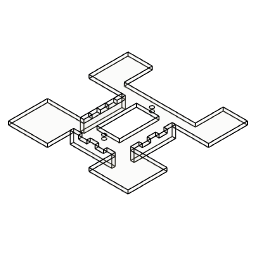
servo support (Autodesk Fusion 360 design; units mm, degrees)
Autodesk Fusion 360 part; units mm, degrees
sketch "Sketch1" plane through (0, 0, 0) normal (0, 0, 1) x (1, 0, 0) in component "main"
  line L0 (-34.5, 34.5) -> (34.5, 34.5)
  line L1 (34.5, 34.5) -> (34.5, -34.5)
  line L2 (34.5, -34.5) -> (-34.5, -34.5)
  line L3 (-34.5, -34.5) -> (-34.5, 34.5)
  line L4 (-34.5, 34.5) -> (34.5, -34.5) construction
  line L5 (34.5, 34.5) -> (-34.5, -34.5) construction
  line L6 (-6.5, 11.375) -> (6.5, 11.375)
  line L7 (6.5, 11.375) -> (6.5, -11.375)
  line L8 (6.5, -11.375) -> (-6.5, -11.375)
  line L9 (-6.5, -11.375) -> (-6.5, 11.375)
  line L10 (-6.5, 11.375) -> (6.5, -11.375) construction
  line L11 (6.5, 11.375) -> (-6.5, -11.375) construction
  dimension "d8" = 69
  dimension "d9" = 13
  dimension "d10" = 22.75
  constraint horizontal L0
  constraint perpendicular L0 L1
  constraint parallel L0 L2
  constraint parallel L1 L3
  constraint coincident L4 origin
  constraint coincident L5 origin
  constraint equal L0 L1
  constraint horizontal L6
  constraint perpendicular L6 L7
  constraint parallel L6 L8
  constraint parallel L7 L9
  constraint coincident L10 origin
  constraint coincident L11 origin
  measures "d8" distance of L0.start L0.end
  measures "d9" distance of L6.start L6.end
  measures "d10" distance of L6.end L7.end
extrude "Extrude1" add sketch "Sketch1" along normal blind 2 makes body 1 in component "main"
sketch "Sketch2" plane through (0, 0, 2) normal (0, 0, 1) x (-1, 0, 0) in component "main"
  line L0 (-6.5, 11.375) -> (6.5, 11.375)
  line L1 (6.5, 11.375) -> (6.5, -11.375)
  line L2 (6.5, -11.375) -> (-6.5, -11.375)
  line L3 (-6.5, -11.375) -> (-6.5, 11.375)
  line L4 (34.5, 34.5) -> (-34.5, 34.5)
  line L5 (-34.5, 34.5) -> (-34.5, -34.5)
  line L6 (-34.5, -34.5) -> (34.5, -34.5)
  line L7 (34.5, -34.5) -> (34.5, 34.5)
  line L8 (-34.5, -12) -> (-15.5, -12)
  line L9 (-15.5, -12) -> (-15.5, 12)
  line L10 (-15.5, 12) -> (-34.5, 12)
  line L11 (-34.5, 12) -> (-34.5, -12)
  line L12 (34.5, -12) -> (15.5, -12)
  line L13 (15.5, -12) -> (15.5, 12)
  line L14 (15.5, 12) -> (34.5, 12)
  line L15 (34.5, 12) -> (34.5, -12)
  line L16 (12, 34.5) -> (-12, 34.5)
  line L17 (-12, 34.5) -> (-12, 21.375)
  line L18 (-12, 21.375) -> (12, 21.375)
  line L19 (12, 21.375) -> (12, 34.5)
  line L20 (20.5, -34.5) -> (-20.5, -34.5)
  line L21 (-20.5, -34.5) -> (-20.5, -18.375)
  line L22 (-20.5, -18.375) -> (20.5, -18.375)
  line L23 (20.5, -18.375) -> (20.5, -34.5)
  dimension "d13" = 24
  dimension "d17" = 10
  dimension "d18" = 9
  dimension "d19" = 14
  dimension "d20" = 7
  constraint horizontal L8
  constraint vertical L9
  constraint horizontal L10
  constraint vertical L11
  constraint horizontal L12
  constraint vertical L13
  constraint horizontal L14
  constraint vertical L15
  constraint horizontal L16
  constraint vertical L17
  constraint horizontal L18
  constraint vertical L19
  constraint midpoint L7 L15
  constraint midpoint L4 L16
  constraint midpoint L5 L11
  constraint equal L9 L18
  constraint equal L13 L18
  constraint equal L8 L12
  constraint horizontal L20
  constraint vertical L21
  constraint horizontal L22
  constraint vertical L23
  constraint midpoint L6 L20
  measures "d13" distance of L17.end L18.end
  measures "d17" distance of L0 L18
  measures "d18" distance of L1 L13
  measures "d19" distance of L7 L23
  measures "d20" distance of L2 L22
extrude "Extrude2" cut sketch "Sketch2" against normal blind 5 contours L4 L16 L17 L18 L19 | L7 L12 L13 L14 L15 | L5 L8 L9 L10 L11 | L6 L20 L21 L22 L23 bodies 1 in component "main"
sketch "Sketch3" plane through (0, 0, 2) normal (0, 0, 1) x (-1, 0, 0) in component "main"
  line L0 (15.5, 12) -> (34.5, 12)
  line L1 (34.5, 12) -> (34.5, 34.5)
  line L2 (34.5, 34.5) -> (12, 34.5)
  line L3 (12, 34.5) -> (12, 21.375)
  line L4 (12, 21.375) -> (-12, 21.375)
  line L5 (-12, 21.375) -> (-12, 34.5)
  line L6 (-12, 34.5) -> (-34.5, 34.5)
  line L7 (-34.5, 34.5) -> (-34.5, 12)
  line L8 (-34.5, 12) -> (-15.5, 12)
  line L9 (-15.5, 12) -> (-15.5, -12)
  line L10 (-15.5, -12) -> (-34.5, -12)
  line L11 (-34.5, -12) -> (-34.5, -34.5)
  line L12 (-34.5, -34.5) -> (-20.5, -34.5)
  line L13 (-20.5, -34.5) -> (-20.5, -18.375)
  line L14 (-20.5, -18.375) -> (20.5, -18.375)
  line L15 (20.5, -18.375) -> (20.5, -34.5)
  line L16 (20.5, -34.5) -> (34.5, -34.5)
  line L17 (34.5, -34.5) -> (34.5, -12)
  line L18 (34.5, -12) -> (15.5, -12)
  line L19 (15.5, -12) -> (15.5, 12)
  line L20 (-6.5, 11.375) -> (6.5, 11.375)
  line L21 (6.5, 11.375) -> (6.5, -11.375)
  line L22 (6.5, -11.375) -> (-6.5, -11.375)
  line L23 (-6.5, -11.375) -> (-6.5, 11.375)
  line L24 (15.5, -12) -> (13.5, -12)
  line L25 (13.5, -12) -> (13.5, -7.2)
  line L26 (13.5, -7.2) -> (15.5, -7.2)
  line L27 (15.5, -7.2) -> (15.5, -12)
  line L28 (13.5, -7.2) -> (15.5, -7.2)
  line L29 (15.5, -7.2) -> (15.5, -2.4)
  line L30 (15.5, -2.4) -> (13.5, -2.4)
  line L31 (13.5, -2.4) -> (13.5, -7.2)
  line L32 (13.5, -2.4) -> (15.5, -2.4)
  line L33 (15.5, -2.4) -> (15.5, 2.4)
  line L34 (15.5, 2.4) -> (13.5, 2.4)
  line L35 (13.5, 2.4) -> (13.5, -2.4)
  line L36 (13.5, 2.4) -> (15.5, 2.4)
  line L37 (15.5, 2.4) -> (15.5, 7.2)
  line L38 (15.5, 7.2) -> (13.5, 7.2)
  line L39 (13.5, 7.2) -> (13.5, 2.4)
  line L40 (13.5, 7.2) -> (15.5, 7.2)
  line L41 (15.5, 7.2) -> (15.5, 12)
  line L42 (15.5, 12) -> (13.5, 12)
  line L43 (13.5, 12) -> (13.5, 7.2)
  line L44 (12, 21.375) -> (7.2, 21.375)
  line L45 (7.2, 21.375) -> (7.2, 19.375)
  line L46 (7.2, 19.375) -> (12, 19.375)
  line L47 (12, 19.375) -> (12, 21.375)
  line L48 (7.2, 19.375) -> (2.4, 19.375)
  line L49 (2.4, 19.375) -> (2.4, 21.375)
  line L50 (2.4, 21.375) -> (7.2, 21.375)
  line L51 (7.2, 21.375) -> (7.2, 19.375)
  line L52 (2.4, 19.375) -> (-2.4, 19.375)
  line L53 (-2.4, 19.375) -> (-2.4, 21.375)
  line L54 (-2.4, 21.375) -> (2.4, 21.375)
  line L55 (2.4, 21.375) -> (2.4, 19.375)
  line L56 (-2.4, 19.375) -> (-7.2, 19.375)
  line L57 (-7.2, 19.375) -> (-7.2, 21.375)
  line L58 (-7.2, 21.375) -> (-2.4, 21.375)
  line L59 (-2.4, 21.375) -> (-2.4, 19.375)
  line L60 (-7.2, 19.375) -> (-12, 19.375)
  line L61 (-12, 19.375) -> (-12, 21.375)
  line L62 (-12, 21.375) -> (-7.2, 21.375)
  line L63 (-7.2, 21.375) -> (-7.2, 19.375)
  line L64 (0, -1.75) -> (0, -22.5)
  line L65 (-13.5, -7.2) -> (-15.5, -7.2)
  line L66 (-13.5, -12) -> (-13.5, -7.2)
  line L67 (-13.5, 7.2) -> (-15.5, 7.2)
  line L68 (-15.5, -2.4) -> (-15.5, 2.4)
  line L69 (-13.5, -2.4) -> (-15.5, -2.4)
  line L70 (-15.5, 7.2) -> (-15.5, 12)
  line L71 (-15.5, -2.4) -> (-13.5, -2.4)
  line L72 (-15.5, -12) -> (-13.5, -12)
  line L73 (-15.5, -7.2) -> (-15.5, -12)
  line L74 (-15.5, 2.4) -> (-13.5, 2.4)
  line L75 (-15.5, 12) -> (-34.5, 12)
  line L76 (-15.5, 7.2) -> (-13.5, 7.2)
  line L77 (-13.5, 2.4) -> (-13.5, -2.4)
  line L78 (-15.5, -7.2) -> (-15.5, -2.4)
  line L79 (-13.5, -2.4) -> (-13.5, -7.2)
  line L80 (-15.5, 12) -> (-13.5, 12)
  line L81 (-13.5, 7.2) -> (-13.5, 2.4)
  line L82 (-15.5, -12) -> (-15.5, 12)
  line L83 (-13.5, -7.2) -> (-15.5, -7.2)
  line L84 (-13.5, 2.4) -> (-15.5, 2.4)
  line L85 (-34.5, -12) -> (-15.5, -12)
  line L86 (-15.5, 2.4) -> (-15.5, 7.2)
  line L87 (-13.5, 12) -> (-13.5, 7.2)
  dimension "d23" = 4.8
  dimension "d24" = 4.8
  dimension "d25" = 4.8
  dimension "d26" = 4.8
  dimension "d27" = 2
  dimension "d28" = 2
  dimension "d29" = 4.8
  dimension "d30" = 4.8
  dimension "d31" = 4.8
  dimension "d32" = 4.8
  dimension "d33" = 4.8
  constraint horizontal L24
  constraint vertical L25
  constraint horizontal L26
  constraint vertical L27
  constraint coincident L18.end L19.start
  constraint horizontal L28
  constraint vertical L29
  constraint horizontal L30
  constraint vertical L31
  constraint coincident L19 L29.end
  constraint horizontal L32
  constraint vertical L33
  constraint horizontal L34
  constraint vertical L35
  constraint coincident L19 L33.end
  constraint horizontal L36
  constraint vertical L37
  constraint horizontal L38
  constraint vertical L39
  constraint coincident L19 L37.end
  constraint horizontal L40
  constraint vertical L41
  constraint horizontal L42
  constraint vertical L43
  constraint coincident L0.start L19.end
  constraint horizontal L44
  constraint vertical L45
  constraint horizontal L46
  constraint vertical L47
  constraint coincident L3.end L4.start
  constraint horizontal L48
  constraint vertical L49
  constraint horizontal L50
  constraint vertical L51
  constraint coincident L4 L49.end
  constraint horizontal L52
  constraint vertical L53
  constraint horizontal L54
  constraint vertical L55
  constraint coincident L4 L53.end
  constraint horizontal L56
  constraint vertical L57
  constraint horizontal L58
  constraint vertical L59
  constraint coincident L4 L57.end
  constraint horizontal L60
  constraint vertical L61
  constraint horizontal L62
  constraint vertical L63
  constraint coincident L4 L5.start
  constraint symmetric L0.start L64 L8.end
  constraint symmetric L0.end L64 L7.end
  constraint symmetric L17.end L64 L10.end
  constraint symmetric L18.end L64 L9.end
  constraint symmetric L24.end L64 L66.start
  constraint symmetric L25.end L64 L65.start
  constraint symmetric L26.end L64 L65.end
  constraint symmetric L29.end L64 L68.start
  constraint symmetric L30.end L64 L69.start
  constraint symmetric L33.end L64 L68.end
  constraint symmetric L34.end L64 L74.end
  constraint symmetric L37.end L64 L67.end
  constraint symmetric L38.end L64 L67.start
  constraint symmetric L42.end L64 L80.end
  measures "d23" distance of L24.end L25.end
  measures "d24" distance of L25.end L30.end
  measures "d25" distance of L30.end L34.end
  measures "d26" distance of L34.end L38.end
  measures "d27" distance of L18.end L24.end
  measures "d28" distance of L3.end L46.end
  measures "d29" distance of L45.end L46.end
  measures "d30" distance of L45.end L48.end
  measures "d31" distance of L48.end L52.end
  measures "d32" distance of L52.end L56.end
  measures "d33" distance of L56.end L60.end
extrude "Extrude3" cut sketch "Sketch3" against normal blind 4 contours L19 L38 L40 L41 L42 L43 | L19 L30 L32 L33 L34 L35 L36 | L4 L44 L45 L46 L47 L51 | L19 L24 L25 L26 L27 L28 | L4 L49 L52 L53 L54 L55 L59 | L4 L57 L60 L61 L62 L63 | L9 L67 L70 L76 L80 L82 L87 | L9 L68 L69 L71 L74 L77 L82 L84 | L9 L65 L66 L72 L73 L82 L83 bodies 1 in component "main"
sketch "Sketch1 (2)" plane through (-13.5, 0, 0) normal (-1, 0, 0) x (0, -1, 0) in component "left slot"
  line L0 (-2.4, 0) -> (2.4, 0)
  line L1 (2.4, 0) -> (2.4, 2)
  line L2 (2.4, 2) -> (-2.4, 2)
  line L3 (-2.4, 2) -> (-2.4, 0)
  line L4 (-12, 2) -> (12, 2)
  line L5 (12, 2) -> (12, -5)
  line L6 (-12, -5) -> (-12, 2)
  line L7 (-12, -5) -> (12, -5)
  point P0 (-12, 2)
  point P1 (12, 2)
  dimension "d36" = 7
  constraint horizontal L4
  constraint vertical L5
  constraint vertical L6
  constraint coincident P0 L4.start
  constraint coincident P1 L4.end
  constraint perpendicular L6 L7
  measures "d36" distance of P1 L5.end
extrude "Extrude1'" add sketch "Sketch1 (2)" along normal blind 2 separate body makes body 2 in component "left slot"
extrude "Extrude1''" add 1 faces at (-15.5, -0.8, -2.6667) along direction (1, 0, 0) blind 2 from surface at 29 separate body on bodies 2 makes body 3 in component "right slot"
sketch "Sketch1 (3)" plane through (0, -19.375, 0) normal (0, -1, 0) x (1, 0, 0) in component "front slot"
  line L0 (-2.4, 0) -> (2.4, 0)
  line L1 (2.4, 0) -> (2.4, 2)
  line L2 (2.4, 2) -> (-2.4, 2)
  line L3 (-2.4, 2) -> (-2.4, 0)
  line L4 (-12, 2) -> (12, 2)
  line L5 (12, 2) -> (12, -5)
  line L6 (12, -5) -> (-12, -5)
  line L7 (-12, -5) -> (-12, 2)
  point P0 (12, 2)
  dimension "d47" = 7
  constraint horizontal L4
  constraint vertical L5
  constraint horizontal L6
  constraint vertical L7
  constraint coincident P0 L4.end
  measures "d47" distance of P0 L5.end
extrude "Extrude1'''" add sketch "Sketch1 (3)" along normal blind 2 separate body makes body 4 in component "front slot"
combine "Combine1" operation cut target body 2 tool bodies 1 keep tools in component "left slot"
combine "Combine1'" operation cut target body 4 tool bodies 1 keep tools in component "front slot"
combine "Combine1''" operation cut target body 3 tool bodies 1 keep tools in component "right slot"
sketch "Sketch4" plane through (0, 0, 2) normal (0, 0, 1) x (-1, 0, 0) in component "main"
  line L0 (-13.5, 7.2) -> (-15.5, 7.2)
  line L1 (-15.5, 7.2) -> (-15.5, 2.4)
  line L2 (-15.5, 2.4) -> (-13.5, 2.4)
  line L3 (-13.5, 2.4) -> (-13.5, -2.4)
  line L4 (-13.5, -2.4) -> (-15.5, -2.4)
  line L5 (-15.5, -2.4) -> (-15.5, -7.2)
  line L6 (-15.5, -7.2) -> (-13.5, -7.2)
  line L7 (-13.5, -7.2) -> (-13.5, -12)
  line L8 (-13.5, -12) -> (-34.5, -12)
  line L9 (-34.5, -12) -> (-34.5, -34.5)
  line L10 (-34.5, -34.5) -> (-20.5, -34.5)
  line L11 (-20.5, -34.5) -> (-20.5, -18.375)
  line L12 (-20.5, -18.375) -> (20.5, -18.375)
  line L13 (20.5, -18.375) -> (20.5, -34.5)
  line L14 (20.5, -34.5) -> (34.5, -34.5)
  line L15 (34.5, -34.5) -> (34.5, -12)
  line L16 (34.5, -12) -> (13.5, -12)
  line L17 (13.5, -12) -> (13.5, -7.2)
  line L18 (13.5, -7.2) -> (15.5, -7.2)
  line L19 (15.5, -7.2) -> (15.5, -2.4)
  line L20 (15.5, -2.4) -> (13.5, -2.4)
  line L21 (13.5, -2.4) -> (13.5, 2.4)
  line L22 (13.5, 2.4) -> (15.5, 2.4)
  line L23 (15.5, 2.4) -> (15.5, 7.2)
  line L24 (15.5, 7.2) -> (13.5, 7.2)
  line L25 (13.5, 7.2) -> (13.5, 12)
  line L26 (13.5, 12) -> (34.5, 12)
  line L27 (34.5, 12) -> (34.5, 34.5)
  line L28 (34.5, 34.5) -> (12, 34.5)
  line L29 (12, 34.5) -> (12, 19.375)
  line L30 (12, 19.375) -> (7.2, 19.375)
  line L31 (7.2, 19.375) -> (7.2, 21.375)
  line L32 (7.2, 21.375) -> (2.4, 21.375)
  line L33 (2.4, 21.375) -> (2.4, 19.375)
  line L34 (2.4, 19.375) -> (-2.4, 19.375)
  line L35 (-2.4, 19.375) -> (-2.4, 21.375)
  line L36 (-2.4, 21.375) -> (-7.2, 21.375)
  line L37 (-7.2, 21.375) -> (-7.2, 19.375)
  line L38 (-7.2, 19.375) -> (-12, 19.375)
  line L39 (-12, 19.375) -> (-12, 34.5)
  line L40 (-12, 34.5) -> (-34.5, 34.5)
  line L41 (-34.5, 34.5) -> (-34.5, 12)
  line L42 (-34.5, 12) -> (-13.5, 12)
  line L43 (-13.5, 12) -> (-13.5, 7.2)
  line L44 (-6.5, 11.375) -> (6.5, 11.375)
  line L45 (6.5, 11.375) -> (6.5, -11.375)
  line L46 (6.5, -11.375) -> (-6.5, -11.375)
  line L47 (-6.5, -11.375) -> (-6.5, 11.375)
  circle A0 centre (0, -13.8) radius 1.1
  line L48 (0, -18.375) -> (0, -11.375) construction
  dimension "d50" = 2.2
  dimension "d51" = 2.425
  constraint midpoint L12 L48.start
  constraint midpoint L46 L48.end
  constraint coincident A0.centre L48
  measures "d50" diameter of A0
  measures "d51" distance of A0.centre L48.end
extrude "Extrude4" cut sketch "Sketch4" against normal blind 6 contours A0 bodies 1 in component "main"
mirror "Mirror1" about plane through (0, 0, 0) normal (0, 1, 0) of "Extrude4" in component "main"
component "main" placed x (1, 0, 0) y (0, 1, 0) z (0, 0, 1) at (0, 0, 0)
component "left slot" placed x (1, 0, 0) y (0, 1, 0) z (0, 0, 1) at (0, 0, 0)
component "right slot" placed x (1, 0, 0) y (0, 1, 0) z (0, 0, 1) at (0, 0, 0)
component "front slot" placed x (1, 0, 0) y (0, 1, 0) z (0, 0, 1) at (0, 0, 0)
equation "Sides = 69 mm"
equation "servolength = 22.75 mm"
equation "servowidth = 13 mm"
equation "thick = 2 mm"
equation "spoutwidth = 30 mm"
equation "servotab = 5 mm"
equation "d8 = Sides"
equation "d9 = servowidth"
equation "d10 = servolength"
equation "d11 = thick"
equation "d13 = slotlength"
equation "spouthole = 15 mm"
equation "offset = 9 mm"
equation "d18 = offset"
equation "d19 = offset + 5 mm"
equation "d20 = servotab + thick"
equation "d23 = slotlength / 5"
equation "d24 = slotlength / 5"
equation "d25 = slotlength / 5"
equation "d26 = slotlength / 5"
equation "d27 = thick"
equation "d28 = thick"
equation "d29 = slotlength / 5"
equation "d30 = slotlength / 5"
equation "d31 = slotlength / 5"
equation "d32 = slotlength / 5"
equation "d33 = slotlength / 5"
equation "d36 = 5 mm + thick"
equation "slotlength = 24 mm"
equation "d39 = thick"
equation "d45 = -thick"
equation "d47 = 5 mm + thick"
equation "d48 = thick"
equation "d51 = 1.325 mm + 1.1 mm"
